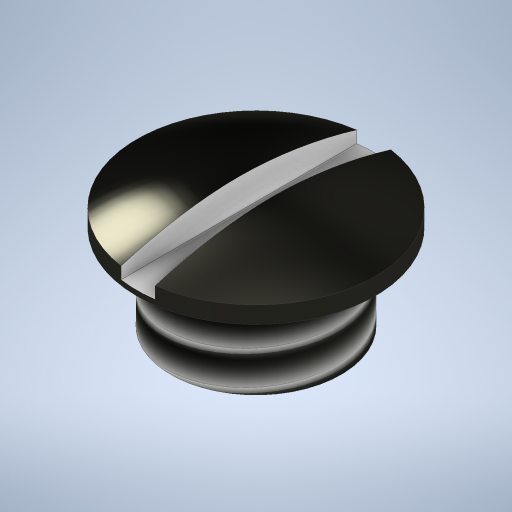
# Autodesk Inventor part: parafusos
Saved by Autodesk Inventor 2023 (Build 270158000, 158)
## iProperties
Created: 2023-08-09
Part Number: parafusos
Material: Genérico
Document SubType Name: Modeling
Designer: azeve
Density: 1 g/cm^3
Appearance: Padrão
Author: azeve
Autodesk Inventor part; units mm, degrees
ref_plane "YZ Plane" through (0, 0, 0) normal (1, 0, 0) x (0, 1, 0)
ref_plane "XZ Plane" through (0, 0, 0) normal (0, 1, 0) x (-1, 0, 0)
sketch "Esboço1" plane through (0, 0, 0) normal (1, 0, 0) x (0, 1, 0)
  line L0 (0, 0) -> (2.5, 0)
  line L1 (2.5, -2.5) -> (2.5, -3.5)
  line L2 (2.5, -3.5) -> (3, -3.5)
  line L3 (2.5, 0) -> (3, 0)
  line L4 (2.5, 0) -> (3.693, 0)
  arc A0 (3, -3.5) -> (3.564, 0) centre (-9.2697, 0.2726) ccw
  line L5 (0, 0) -> (0, -2.5)
  line L6 (0, -2.5) -> (2.5, -2.5)
  dimension "d0" = 2.5
  dimension "d1" = 3.5
  dimension "d3" = 0.5
  dimension "d11" = 2.5
  constraints: 14 end point, 4 perpendicular, 2 horizontal, 2 point on circle, 1 centre point, 1 point on line, 1 vertical
  measures "d0" distance of L0.start L0.end
  measures "d1" distance of L0.end L1.end
  measures "d3" distance of L0.end L3.end
  measures "d11" distance of L0.start L5.end
revolve "Revolução1" add sketch "Esboço1" angle 360 about axis through (0, 0, 0) along (0, 1, 0)
thread "Rosca1" size "M6x1" class "6g" standard "ANSI Metric M Profile" full length
ref_plane "Plano de trabalho1" through (0, 4.25, 0) normal (0, -1, 0) x (1, 0, 0)
sketch "Esboço2" plane through (0, 4.25, 0) normal (0, -1, 0) x (1, 0, 0)
  line L0 (-0.5012, 4.0955) -> (0.5012, 4.0955)
  line L1 (0.5012, 4.0955) -> (0.5012, -4.0955)
  line L2 (0.5012, -4.0955) -> (-0.5012, -4.0955)
  line L3 (-0.5012, -4.0955) -> (-0.5012, 4.0955)
  line L4 (-0.5012, 4.0955) -> (0.5012, -4.0955) construction
  line L5 (0.5012, 4.0955) -> (-0.5012, -4.0955) construction
  point P0 (0, 0)
  constraints: 12 end point, 2 midpoint, 2 parallel, 1 horizontal, 1 perpendicular
extrude "Extrusão1" cut sketch "Esboço2" along normal blind 1.6
